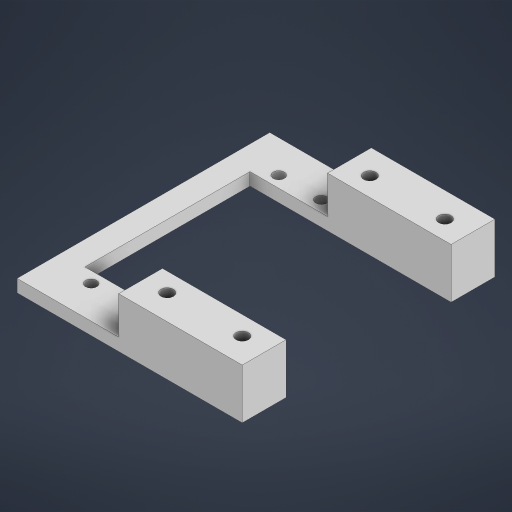
# Autodesk Inventor part: Servo_fix
Saved by Autodesk Inventor 2023 (Build 270158000, 158)
## iProperties
Created: 2023-11-05
Part Number: Servo_fix
Material: Generic
Document SubType Name: Modeling
Designer: Abhinav
Density: 1 g/cm^3
Appearance: Default
Author: Abhinav
Autodesk Inventor part; units mm, degrees
ref_plane "YZ Plane" through (0, 0, 0) normal (1, 0, 0) x (0, 1, 0)
ref_plane "XZ Plane" through (0, 0, 0) normal (0, 1, 0) x (-1, 0, 0)
ref_plane "XY Plane" through (0, 0, 0) normal (0, 0, 1) x (1, 0, 0)
sketch "Sketch1" plane through (0, 0, 0) normal (0, 1, 0) x (-1, 0, 0)
  line L0 (8.5, -37.5) -> (8.5, 37.5) construction
  line L1 (-8.5, 37.5) -> (-8.5, -37.5) construction
  line L2 (15.5, 33) -> (15.5, -33)
  line L3 (-15.5, -33) -> (-15.5, 33) construction
  line L4 (15.5, -33) -> (-15.5, -33)
  line L5 (-8.5, -37.5) -> (8.5, -37.5) construction
  circle A0 centre (8.5, -37.5) radius 2.25
  line L6 (0, -37.5) -> (-8.5, -37.5) construction
  circle A1 centre (-8.5, -37.5) radius 2.25
  line L7 (-15.5, 33) -> (15.5, 33)
  circle A2 centre (-8.5, 37.5) radius 2.25
  line L8 (8.5, 37.5) -> (-8.5, 37.5) construction
  circle A3 centre (8.5, 37.5) radius 2.25
  line L9 (-15.5, -33) -> (15.5, 33) construction
  line L10 (0, 33) -> (0, 19.5) construction
  line L11 (0, 0) -> (15.5, 0) construction
  line L12 (0, 19.5) -> (-39.9, 19.5) construction
  line L13 (-54.9, -40.5) -> (-24.9, -40.5) construction
  circle A4 centre (-54.9, -40.5) radius 2.5
  circle A5 centre (-24.9, -40.5) radius 2.5
  line L14 (-24.9, -40.5) -> (-24.9, -50.5) construction
  line L15 (25.1, 50.5) -> (25.1, -50.5)
  line L16 (25.1, -50.5) -> (-24.9, -50.5)
  line L17 (-15.5, -33) -> (-64.9, -33)
  line L18 (-64.9, -50.5) -> (-24.9, -50.5)
  line L19 (0, 0) -> (-54.9, 0) construction
  line L20 (-54.9, 40.5) -> (-24.9, 40.5) construction
  circle A6 centre (-54.9, 40.5) radius 2.5
  circle A7 centre (-24.9, 40.5) radius 2.5
  line L21 (-24.9, 40.5) -> (-24.9, 50.5) construction
  line L22 (-15.5, 33) -> (-64.9, 33)
  line L23 (-64.9, 50.5) -> (25.1, 50.5)
  line L24 (-24.9, 40.5) -> (-54.9, -40.5)
  circle A8 centre (-39.9, 19.5) radius 3.9303 construction
  line L25 (-15.5, -50.5) -> (-15.5, -33)
  line L26 (-15.5, 33) -> (-15.5, 50.5)
  line L27 (-64.9, -50.5) -> (-64.9, -33)
  line L28 (-64.9, 33) -> (-64.9, 50.5)
  point P0 (0, 0)
  point P1 (8.5, 33)
  dimension "d0" = 8.5
  dimension "d1" = 4.5
  dimension "d2" = 17
  dimension "d3" = 75
  dimension "d4" = 31
  dimension "d9" = 13.5
  dimension "d13" = 39.9
  dimension "d14" = 30
  dimension "d18" = 10
  constraints: 58 end point, 9 centre point, 9 coincident, 5 perpendicular, 5 point on line, 5 symmetric about line, 4 equal radius, 4 parallel, 3 midpoint, 2 vertical, 2 other
  measures "d0" distance of L6.start L6.end
  measures "d1" diameter of A1
  measures "d2" distance of L1.start L0.end
  measures "d3" distance of L0.end L5.end
  measures "d4" distance of L3.end L2.start
  measures "d9" distance of L10.start L10.end
  measures "d13" distance of L10.end L12.end
  measures "d14" distance of L13.end L13.start
  measures "d18" distance of L14.start L14.end
extrude "Extrusion1" add sketch "Sketch1" along normal blind 5 contours L7 L26 L23 L15 L16 L25 L4 L2
extrude "Extrusion2" add sketch "Sketch1" along normal blind 20 contours L22 L28 L23 L26 | L25 L16 L18 L27 L17
body "Solid1"
